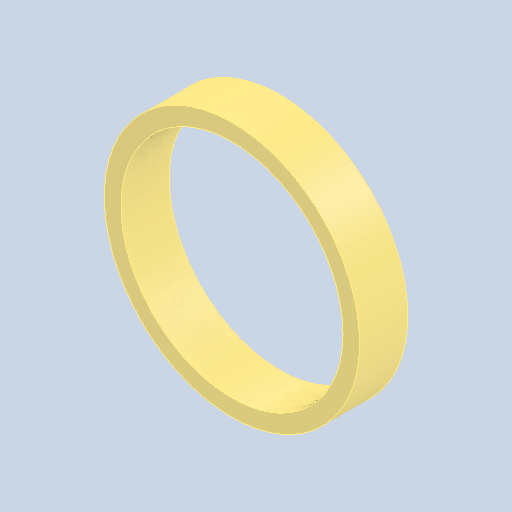
# Autodesk Inventor part: TH22_Urethane_roller_sn
Saved by Autodesk Inventor 2025.1 (Build 291241000, 241)
## iProperties
Created: 2021-11-15
Part Number: TH22_Urethane_roller_sn
Material: ポリスチレン
Document SubType Name: Modeling
Designer: 中島 青蔵
Density: 1.021 g/cm^3
Appearance: 光沢 - ゴールド
Author: 中島 青蔵
Autodesk Inventor part; units mm, degrees
ref_plane "YZ Plane" through (0, 0, 0) normal (1, 0, 0) x (0, 1, 0)
ref_plane "XZ Plane" through (0, 0, 0) normal (0, 1, 0) x (-1, 0, 0)
ref_plane "XY Plane" through (0, 0, 0) normal (0, 0, 1) x (1, 0, 0)
sketch "スケッチ1" plane through (0, 0, 0) normal (0, 0, 1) x (1, 0, 0)
  circle A0 centre (0, 0) radius 67
  circle A1 centre (0, 0) radius 77
  dimension "d0" = 134
  dimension "d1" = 154
  constraints: 2 centre point, 2 coincident
  measures "d0" diameter of A0
  measures "d1" diameter of A1
extrude "押し出し1" add sketch "スケッチ1" along normal blind 29
